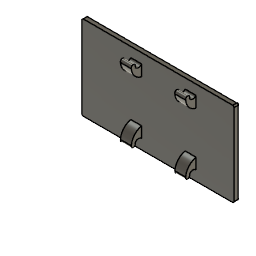
imu_box_v2 (Autodesk Fusion 360 design; units mm, degrees)
Autodesk Fusion 360 part; units mm, degrees
note: some values were not read from the file. Set by a fixed rule: which sketch regions a step uses.
sketch "Sketch1" plane through (0, 0, 0) normal (0, 1, 0) x (1, 0, 0)
  line L0 (0, 0) -> (50, 0)
  line L1 (50, 0) -> (50, -25)
  line L2 (50, -25) -> (0, -25)
  line L3 (0, -25) -> (0, 0)
  line L4 (53, 3) -> (53, -28)
  line L5 (53, -28) -> (-3, -28)
  line L6 (-3, -28) -> (-3, 3)
  line L7 (-3, 3) -> (53, 3)
  dimension "d1" = 50
  dimension "d2" = 25
  dimension "d3" = -3
  constraint horizontal L0
  constraint vertical L1
  constraint horizontal L2
  constraint vertical L3
  constraint coincident L0.start L3.end
  measures "d1" distance of L1.end L2.end
  measures "d2" distance of L0.end L1.end
extrude "Extrude1" add sketch "Sketch1" along normal blind 25 makes body 1
extrude "Extrude2" add sketch "Sketch1" along normal blind 3 contours L0 L1 L2 L3 bodies 1
ref_plane "WorkPlane1" through (25, 14, 12.5) normal (0, 0, 1) x (1, 0, 0)
ref_plane "WorkPlane2" through (25, 14, 12.5) normal (1, 0, 0) x (0, 0, -1)
sketch "Sketch3" plane through (25, 0, 0) normal (1, 0, 0) x (0, 1, 0)
  line L0 (25, 28) -> (0, 28)
  line L1 (0, 28) -> (0, -3)
  line L2 (0, -3) -> (25, -3)
  line L3 (25, -3) -> (25, 0)
  line L4 (25, 0) -> (3, 0)
  line L5 (3, 0) -> (3, 25)
  line L6 (3, 25) -> (25, 25)
  line L7 (25, 25) -> (25, 28)
  circle A0 centre (21.9321, 25) radius 0.75
  circle A1 centre (21.9321, 25) radius 0.85
  line L8 (25, -3) -> (27, -3)
  line L9 (27, -3) -> (27, 28)
  line L10 (27, 28) -> (25, 28)
  line L11 (25, 25) -> (25, 0)
  arc A2 (21.2162, 24.7762) -> (25, 20.3) centre (26.0741, 25.0452) ccw
  arc A3 (22.8, 24.3) -> (25, 24.3884) centre (23.869, 25.1154) ccw
  arc A4 (22.666, 24.8456) -> (22.8, 24.3) centre (23.3593, 24.7266) ccw
  line L12 (27.2, 12.5) -> (0.8, 12.5)
  arc A5 (25, 0.6116) -> (22.8, 0.7) centre (23.869, -0.1154) ccw
  arc A6 (22.8, 0.7) -> (22.666, 0.1544) centre (23.3593, 0.2734) ccw
  arc A7 (25, 4.7) -> (21.2162, 0.2238) centre (26.0741, -0.0452) ccw
  circle A8 centre (21.9321, 0) radius 0.85
  circle A9 centre (21.9321, 0) radius 0.75
  dimension "d8" = 1.5
  dimension "d9" = 0.1
  constraint coincident L6 A0.centre
  constraint coincident L2.end L3.start
  constraint perpendicular L3 L8
  constraint perpendicular L8 L9
  constraint coincident L0.start L7.end
  constraint coincident L6.end L7.start
  constraint coincident L3.end L4.start
  constraint coincident L11 A2.end
  constraint coincident L11 A3.end
  constraint coincident A0 A4.start
  constraint tangent A3 A4
  constraint symmetric A0 L12 A9
  constraint symmetric A1 L12 A8
  constraint symmetric A2.end L12 A7.start
  constraint symmetric A2 L12 A7
  constraint symmetric A3.end L12 A5.start
  constraint symmetric A3 L12 A5
  constraint symmetric A3.start L12 A5.end
  constraint symmetric A4.start L12 A6.end
  constraint symmetric A4 L12 A6
  constraint symmetric A2.start L12 A7.end
  constraint coincident A0 A2.start
  measures "d8" diameter of A0
extrude "Extrude3" cut sketch "Sketch3" against normal up to surface (50 mm away) from surface at 25 contours L6 A0 A1 A4 | L6 A0 A1 | L6 A0 | L6 A0 | L4 A8 A9 | L4 A6 A8 A9 | L4 A9 | L4 A9 bodies 1
extrude "Extrude4" add sketch "Sketch3" along normal mid plane 56 separate body contours L7 L9 L10 L11 L12 | L3 L8 L9 L11 L12 makes body 2
extrude "Extrude5" add sketch "Sketch3" along normal blind 4 from surface at 10 contours A1 L11 A2 A3 A4 | L6 A0 | L6 A0 | A0 A1 A2 A4 | L11 A5 A6 A7 A8 | A6 A7 A8 A9 | L4 A9 | L4 A9 bodies 2
extrude "Extrude6" add sketch "Sketch3" along normal blind 4 from surface at -10 contours A1 L11 A2 A3 A4 | L6 A0 | L6 A0 | A0 A1 A2 A4 | L11 A5 A6 A7 A8 | A6 A7 A8 A9 | L4 A9 | L4 A9 bodies 2
fillet "Fillet1" radius 1 2 edges at (25, 22.7821, 25) (25, 22.7821, 0) on bodies 1
fillet "Fillet2" radius 1 2 edges at (25, 25, 0) (25, 25, 25) on bodies 1
fillet "Fillet2" radius 0.5 2 edges at (50, 25, 12.5) (0, 25, 12.5) on bodies 1
fillet "Fillet3" radius 0.5 4 edges at (25, 27, 28) (25, 27, -3) (-3, 27, 12.5) (53, 27, 12.5) on bodies 2
fillet "Fillet4" radius 0.5 16 edges at (53, 12.5, -3) (53, 12.5, 28) (-3, 12.5, -3) (-3, 12.5, 28) (-3, 0, 12.5) (25, 0, -3) (53, 0, 12.5) (25, 0, 28) (53, 25.75, -3) (52.8536, 26.8536, -2.8536) (52.8536, 26.8536, 27.8536) (53, 25.75, 28) (-2.8536, 26.8536, -2.8536) (-3, 25.75, -3) (-3, 25.75, 28) (-2.8536, 26.8536, 27.8536) on bodies 1 2
hidden bodies 1
